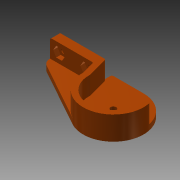
# Autodesk Inventor part: z pulley holder
Saved by Autodesk Inventor 2013 (Build 170138000, 138)
## iProperties
Created: 2014-01-26
Part Number: z pulley holder
Material: Generic
Document SubType Name: Modeling
Designer: employee
Density: 1 g/cm^3
Author: employee
Autodesk Inventor part; units mm, degrees
ref_plane "YZ Plane" through (0, 0, 0) normal (1, 0, 0) x (0, 1, 0)
ref_plane "XZ Plane" through (0, 0, 0) normal (0, 1, 0) x (-1, 0, 0)
ref_plane "XY Plane" through (0, 0, 0) normal (0, 0, 1) x (1, 0, 0)
sketch "Sketch1" plane through (0, 0, 0) normal (0, 0, 1) x (1, 0, 0)
  circle A0 centre (0, 0) radius 13.165 construction
  line L0 (-42.5, 12.5) -> (-22.5, 12.5) construction
  line L1 (-42.5, 12.5) -> (-17.5, 12.5)
  line L2 (-17.5, 12.5) -> (-17.5, 16.665)
  line L3 (-17.5, 16.665) -> (0, 16.665)
  arc A1 (-8.0971, -14.5657) -> (0, 16.665) centre (0, 0) ccw
  line L4 (-8.0971, -14.5657) -> (-39.9294, 3.1299)
  arc A2 (-42.5, 7.5) -> (-39.9294, 3.1299) centre (-37.5, 7.5) ccw
  line L5 (-42.5, 7.5) -> (-42.5, 12.5)
  dimension "d0" = 26.33
  dimension "d2" = 12.5
  dimension "d3" = 22.5
  dimension "d4" = 20
  dimension "d5" = 25
  dimension "d6" = 5
  dimension "d8" = 3.5
  dimension "d9" = 5
  constraints: 12 end point, 4 point on circle, 4 tangent, 3 centre point, 2 coincident, 2 perpendicular, 1 horizontal, 1 parallel, 1 point on line
  measures "d0" diameter of A0
  measures "d2" distance from line of L0 point (0, 0)
  measures "d3" horizontal distance of L0.end point (0, 0)
  measures "d4" distance of L0.start L0.end
  measures "d5" distance of L0.start L1.end
  measures "d6" radius of A2
  measures "d8" radial gap between concentric circles of A0 A1
  measures "d9" distance of L5.start L0.start
extrude "Extrusion1" add sketch "Sketch1" along normal blind 3
sketch "Sketch2" plane through (0, 0, 3) normal (0, 0, 1) x (1, 0, 0)
  arc A0 (-8.0971, -14.5657) -> (0, 16.665) centre (0, 0) ccw projected
  line L0 (0, 16.665) -> (-17.5, 16.665) projected
  line L1 (-42.5, 12.5) -> (-17.5, 12.5)
  line L2 (-17.5, 12.5) -> (-17.5, 7.5)
  line L3 (-17.5, 7.5) -> (-42.5, 7.5)
  line L4 (-42.5, 7.5) -> (-42.5, 12.5)
  circle A1 centre (0, 0) radius 13.665
  arc A2 (-16.665, 0) -> (0, 16.665) centre (0, 0) ccw
  line L5 (-16.665, 0) -> (-16.665, 7.5)
  line L6 (-16.665, 7.5) -> (-17.5, 7.5)
  line L7 (-17.5, 7.5) -> (-17.5, 16.665)
  dimension "d12" = 5
  dimension "d14" = 27.33
  constraints: 15 end point, 3 coincident, 3 parallel, 2 centre point, 2 perpendicular, 2 point on circle, 1 collinear, 1 concentric, 1 horizontal, 1 tangent
  measures "d12" distance between parallel lines of L1 L3
  measures "d14" diameter of A1
extrude "Extrusion2" add sketch "Sketch2" along normal blind 10
sketch "Sketch3" plane through (0, 0, 13) normal (0, 0, 1) x (1, 0, 0)
  arc A0 (-16.665, 0) -> (0, 16.665) centre (0, 0) ccw projected
  arc A1 (-12.557, -3.3646) -> (12.557, -3.3646) centre (0, 0) ccw
  line L0 (-17.924, 16.665) -> (-12.557, -3.3646)
  line L1 (17.924, 16.665) -> (12.557, -3.3646)
  line L2 (-17.924, 16.665) -> (17.924, 16.665)
  dimension "d17" = 26
  dimension "d19" = 30
  constraints: 6 end point, 2 horizontal alignment, 2 point on circle, 2 tangent, 1 centre point, 1 coincident, 1 horizontal
  measures "d17" diameter of A1
  measures "d19" angle of L0 L1
extrude "Extrusion3" cut sketch "Sketch3" against normal blind 10
sketch "Sketch4" plane through (0, 0, 13) normal (0, 0, 1) x (1, 0, 0)
  line L0 (-13.6469, 0.7028) -> (-17.5, 15.0827) projected
  line L1 (-42.5, 7.5) -> (-16.665, 7.5) projected
  line L2 (-16.665, 7.5) -> (-16.665, 0) projected
  line L3 (-17.5, 12.5) -> (-16.808, 12.5)
  line L4 (-18.574, 7.5) -> (-16.665, 0.3754)
  dimension "d23" = 3
  constraints: 4 end point, 3 point on line, 1 parallel, 1 perpendicular
  measures "d23" distance between parallel lines of L0 L4
extrude "Extrusion4" add sketch "Sketch4" against normal up to surface (10 mm away)
sketch "Sketch5" plane through (0, 0, 13) normal (0, 0, 1) x (1, 0, 0)
  line L0 (-13.6469, 0.7028) -> (-17.5, 15.0827) projected
  line L1 (-17.5, 15.0827) -> (-17.5, 12.5) projected
  line L2 (-16.665, 0.3754) -> (-16.665, 0) projected
  line L3 (-17.5, 12.5) -> (-16.808, 12.5)
  constraints: 2 end point, 1 perpendicular, 1 point on line
extrude "Extrusion5" cut sketch "Sketch5" against normal up to surface (10 mm away)
fillet "Fillet1" radius 1 8 edges at (15.2557, 6.7071, 8) (-17.5, 16.665, 1.5) (-16.665, 0.3754, 8) (-18.574, 7.5, 8) (-42.5, 10, 13) (-13.6469, 0.7028, 8) (-16.808, 12.5, 8) (13.6469, 0.7028, 8)
sketch "Sketch6" plane through (0, 0, 3) normal (0, 0, 1) x (1, 0, 0)
  arc A0 (16.3213, 3.3671) -> (0, 16.665) centre (0, 0) ccw projected
  circle A1 centre (0, 0) radius 1.55
  dimension "d29" = 3.1
  constraints: 1 centre point, 1 coincident
  measures "d29" diameter of A1
extrude "Extrusion6" cut sketch "Sketch6" against normal blind 2.1
sketch "Sketch7" plane through (0, 0, 0) normal (0, 0, -1) x (-1, 0, 0)
  arc A0 (0, 16.665) -> (8.0971, -14.5657) centre (0, 0) ccw projected
  line L0 (3.2332, 0) -> (1.6166, -2.8)
  line L1 (1.6166, -2.8) -> (-1.6166, -2.8)
  line L2 (-1.6166, -2.8) -> (-3.2332, 0)
  line L3 (-3.2332, 0) -> (-1.6166, 2.8)
  line L4 (-1.6166, 2.8) -> (1.6166, 2.8)
  line L5 (1.6166, 2.8) -> (3.2332, 0)
  dimension "d33" = 5.6
  constraints: 12 end point, 1 coincident, 1 horizontal, 13 other
  measures "d33" distance between parallel lines of L1 L4
extrude "Extrusion7" cut sketch "Sketch7" against normal blind 2.5
sketch "Sketch8" plane through (-42.5, 7.5, 3) normal (0, -1, 0) x (1, 0, 0)
  line L0 (0, 0) -> (0, 9) projected
  line L1 (23.1586, 10) -> (23.1586, 0) projected
  line L2 (1, 10) -> (23.1586, 10) projected
  line L3 (5, 5) -> (20, 5)
  circle A0 centre (5, 5) radius 1.55
  circle A1 centre (20, 5) radius 1.55
  point P0 (42.5, -3)
  point P1 (23.1586, 5)
  dimension "d36" = 5
  dimension "d37" = 15
  dimension "d38" = 3.1
  constraints: 2 centre point, 2 coincident, 2 end point, 1 equal radius, 1 horizontal alignment, 1 midpoint, 1 parallel
  measures "d36" distance from line of L0 L3.start
  measures "d37" distance of L3.start L3.end
  measures "d38" diameter of A0
extrude "Extrusion8" cut sketch "Sketch8" against normal through all
sketch "Sketch9" plane through (-42.5, 7.5, 3) normal (0, -1, 0) x (1, 0, 0)
  circle A0 centre (5, 5) radius 1.55 projected
  circle A1 centre (20, 5) radius 1.55 projected
  line L0 (6.6166, 7.8) -> (8.2332, 5)
  line L1 (8.2332, 5) -> (6.6166, 2.2)
  line L2 (6.6166, 2.2) -> (3.3834, 2.2)
  line L3 (3.3834, 2.2) -> (1.7668, 5)
  line L4 (1.7668, 5) -> (3.3834, 7.8)
  line L5 (3.3834, 7.8) -> (6.6166, 7.8)
  line L6 (16.7668, 5) -> (18.3834, 7.8)
  line L7 (18.3834, 7.8) -> (21.6166, 7.8)
  line L8 (21.6166, 7.8) -> (23.2332, 5)
  line L9 (23.2332, 5) -> (21.6166, 2.2)
  line L10 (21.6166, 2.2) -> (18.3834, 2.2)
  line L11 (18.3834, 2.2) -> (16.7668, 5)
  point P0 (42.5, -3)
  dimension "d41" = 5.6
  constraints: 24 end point, 2 coincident, 2 horizontal, 1 collinear, 26 other
  measures "d41" distance between parallel lines of L2 L5
extrude "Extrusion9" cut sketch "Sketch9" along normal mid plane 5
sketch "Sketch10" plane through (0, 0, 3) normal (0, 0, 1) x (1, 0, 0)
  circle A0 centre (0, 0) radius 1.55 projected
  arc A1 (16.3213, 3.3671) -> (0, 16.665) centre (0, 0) ccw projected
  circle A2 centre (0, 0) radius 7.5
  dimension "d44" = 15
  constraints: 1 centre point, 1 coincident
  measures "d44" diameter of A2
extrude "Extrusion10" add sketch "Sketch10" along normal blind 1
body "Solid1"
